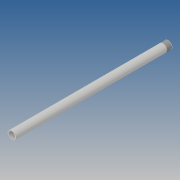
# Autodesk Inventor part: pre_barrel
Saved by Autodesk Inventor 2019 (Build 230136000, 136)
## iProperties
Created: 2019-03-08
Part Number: pre_barrel
Material: Générique
Document SubType Name: Modeling
Designer: Theo
Density: 1 g/cm^3
Appearance: Par défaut
Author: Theo
Autodesk Inventor part; units mm, degrees
ref_plane "YZ Plane" through (0, 0, 0) normal (1, 0, 0) x (0, 1, 0)
ref_plane "XZ Plane" through (0, 0, 0) normal (0, 1, 0) x (-1, 0, 0)
ref_plane "XY Plane" through (0, 0, 0) normal (0, 0, 1) x (1, 0, 0)
sketch "Esquisse1" plane through (0, 0, 0) normal (1, 0, 0) x (0, 1, 0)
  line L0 (0, 0) -> (0, 91.9394)
  line L1 (6.25, 300) -> (6.25, 0)
  line L2 (6.25, 0) -> (7.75, 0)
  line L3 (7.75, 0) -> (7.75, 300)
  line L4 (7.75, 300) -> (6.25, 300)
  dimension "d5" = 12.5
  dimension "d6" = 15.5
  dimension "d7" = 300
  constraints: 10 end point, 2 horizontal, 2 vertical, 1 horizontal alignment, 1 parallel
  measures "d5" diameter of L1 L0
  measures "d6" diameter of L3 L0
  measures "d7" distance of L2.end L3.end
revolve "Révolution1" add sketch "Esquisse1" angle 360 about axis through (0, 0, 0) along (0, 0, 1)
thread "Filetage1" size "M16x1.5" class "6g" standard "ISO Metric profile" length 10
